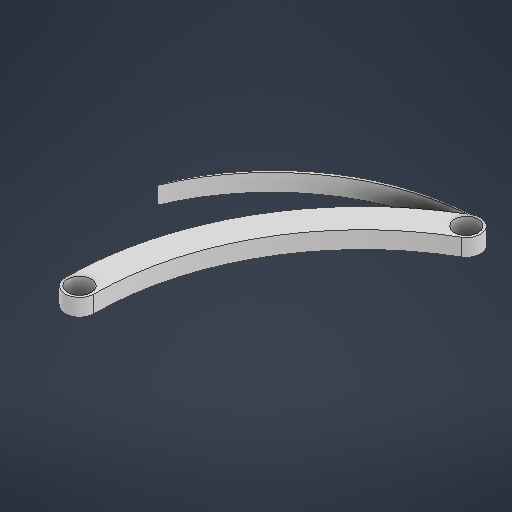
# Autodesk Inventor part: Aparatus_Connector_2
Saved by Autodesk Inventor 2026.2 (Build 302298000, 298)
## iProperties
Created: 2025-12-30
Part Number: Aparatus_Connector_2
Material: Generic
Document SubType Name: Modeling
Designer: Cobble
Density: 1 g/cm^3
Appearance: Default
Author: Cobble
Autodesk Inventor part; units mm, degrees
ref_plane "YZ Plane" through (0, 0, 0) normal (1, 0, 0) x (0, 1, 0)
ref_plane "XZ Plane" through (0, 0, 0) normal (0, 1, 0) x (-1, 0, 0)
ref_plane "XY Plane" through (0, 0, 0) normal (0, 0, 1) x (1, 0, 0)
sketch "Sketch1" plane through (0, 0, 0) normal (0, 0, 1) x (1, 0, 0)
  circle A0 centre (0, 0) radius 99.25 construction
  circle A1 centre (-99.25, 0) radius 4.15
  arc A2 (-49.625, 85.953) -> (-99.25, 0) centre (0, 0) ccw
  line L0 (0, 0) -> (-49.625, 85.953) construction
  line L1 (0, 0) -> (-99.25, 0) construction
  circle A3 centre (-49.625, 85.953) radius 4.15
  circle A4 centre (0, 0) radius 95.25 construction
  circle A5 centre (0, 0) radius 103.25 construction
  circle A6 centre (-49.625, 85.953) radius 5
  circle A7 centre (-99.25, 0) radius 5
  circle A8 centre (0, 0) radius 94.25
  circle A9 centre (0, 0) radius 104.25
  line L2 (-99.25, 0) -> (-49.625, 85.953) construction
  line L3 (-99.25, 0) -> (0, 0) construction
  arc A10 (0, 0) -> (-10.8176, 45.0586) centre (-99.25, 0) ccw
  line L4 (-99.25, 0) -> (-10.8176, 45.0586) construction
  line L5 (-99.25, 0) -> (0, 0) construction
  circle A11 centre (-10.8176, 45.0586) radius 105.3
  arc A12 (-52.125, 90.2831) -> (-116.1176, 45.0586) centre (-48.9244, 17.8674) ccw
  line L6 (-52.125, 90.2831) -> (-52.9886, 89.779)
  line L7 (-116.1176, 45.0586) -> (-116.1129, 44.0586)
  arc A13 (-52.9886, 89.779) -> (-116.1129, 44.0586) centre (-46.9619, 15.0215) ccw
  point P0 (-94.25, 0)
  point P1 (-47.125, 81.6229)
  point P2 (-104.25, 0)
  dimension "d0" = 198.5
  dimension "d4" = 10
  dimension "d1" = 8.3
  dimension "d2" = 60
  dimension "d3" = 8.3
  dimension "d5" = 10
  dimension "d9" = 60
  dimension "d10" = 27
  dimension "d11" = 210.6
  dimension "d12" = 1
  dimension "d13" = 1
  dimension "d14" = 75
  constraints: 16 end point, 12 centre point, 12 point on circle, 11 coincident, 2 tangent, 1 horizontal alignment, 1 point on line, 5 other
  measures "d1" diameter of A1
  measures "d2" angle of L0 L1
  measures "d3" diameter of A3
  measures "d5" diameter of A7
  measures "d9" angle of L3 L2
  measures "d10" angle of L5 L4
  measures "d11" diameter of A11
  measures "d12" distance of L6.start L6.end
  measures "d13" distance of L7.start L7.end
  measures "d14" radius of A13
extrude "Extrusion1" add sketch "Sketch1" along normal blind 6 contours A6 A8 A7 A2 | A2 A7 A9 A6 | A6 | A7 | A9 A13 A11 A12
body "Solid1"
